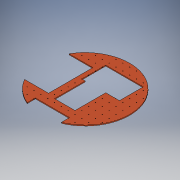
# Autodesk Inventor part: existing copper plate 1
Saved by Autodesk Inventor 2018 (Build 220112000, 112)
## iProperties
Created: 2018-11-02
Part Number: existing copper plate 1
Material: Copper
Document SubType Name: Modeling
Designer: freyja
Mass: 1197.4 g
Surface Area: 917.652 cm^2
Volume: 133.937 cm^3
Density: 8.94 g/cm^3
Appearance: Copper - Satin
Author: freyja
Autodesk Inventor part; units mm, degrees
ref_plane "YZ Plane" through (0, 0, 0) normal (1, 0, 0) x (0, 1, 0)
ref_plane "XZ Plane" through (0, 0, 0) normal (0, 1, 0) x (-1, 0, 0)
ref_plane "XY Plane" through (0, 0, 0) normal (0, 0, 1) x (1, 0, 0)
sketch "Sketch1" plane through (0, 0, 0) normal (0, 1, 0) x (-1, 0, 0)
  circle A0 centre (0, 0) radius 165.1
  dimension "d0" = 330.2
  constraints: 1 centre point, 1 coincident
  measures "d0" diameter of A0
extrude "Extrusion1" add sketch "Sketch1" along normal blind 3.175
sketch "Sketch2" plane through (0, 3.175, 0) normal (0, 1, 0) x (1, 0, 0)
  line L0 (0, 0) -> (-12.7, 0)
  line L1 (0, 0) -> (12.7, 0) construction
  circle A0 centre (0, 0) radius 165.1 projected
  dimension "d34" = 12.7
  dimension "d35" = 180
  constraints: 4 end point, 3 coincident, 2 horizontal, 1 collinear
  measures "d34" distance of L0.start L0.end
  measures "d35" angle of L0 L1
hole "Hole1" at (-12.7, 3.175, 0) direction (0, -1, 0) diameter 2.159 end through all
pattern_linear "Rectangular Pattern1" count 13 spacing 25.4 along (1, 0, 0) count 13 spacing 25.4 along (0, 0, 1) of "Hole1" first direction both ways yes second direction both ways yes
sketch "Sketch3" plane through (0, 3.175, 0) normal (0, 1, 0) x (1, 0, 0)
  circle A0 centre (0, 0) radius 165.1 projected
  line L0 (165.1, 0) -> (50.8, 0) construction
  line L1 (50.8, -88.9) -> (-25.4, -88.9)
  line L2 (-25.4, -88.9) -> (-25.4, 114.3)
  line L3 (-25.4, 114.3) -> (50.8, 114.3)
  line L4 (50.8, 114.3) -> (50.8, -88.9)
  line L5 (50.8, -88.9) -> (-25.4, 114.3) construction
  line L6 (-25.4, -88.9) -> (50.8, 114.3) construction
  line L7 (0, 165.1) -> (0, 114.3) construction
  line L8 (101.6, 25.4) -> (-38.1, 25.4)
  line L9 (-38.1, 25.4) -> (-38.1, 114.3)
  line L10 (-38.1, 114.3) -> (101.6, 114.3)
  line L11 (101.6, 114.3) -> (101.6, 25.4)
  line L12 (-25.4, 114.3) -> (-38.1, 114.3) construction
  line L13 (-25.4, -88.9) -> (-25.4, -121.92) construction
  line L14 (-63.5, -198.12) -> (63.5, -198.12)
  line L15 (63.5, -198.12) -> (63.5, -121.92)
  line L16 (63.5, -121.92) -> (-63.5, -121.92)
  line L17 (-63.5, -121.92) -> (-63.5, -198.12)
  line L18 (0, 0) -> (0, -165.1) construction
  line L19 (0, -198.12) -> (0, -121.92)
  line L20 (-181.0808, -82.55) -> (-181.0808, 82.55)
  line L21 (-181.0808, 82.55) -> (-54.0808, 82.55)
  line L22 (-54.0808, 82.55) -> (-54.0808, -82.55)
  line L23 (-54.0808, -82.55) -> (-181.0808, -82.55)
  line L24 (-142.9808, 82.55) -> (-54.0808, 82.55)
  circle A1 centre (0, 0) radius 165.1 projected
  line L25 (-142.9808, -82.55) -> (-54.0808, -82.55)
  point P0 (12.7, 12.7)
  dimension "d16" = 114.3
  dimension "d17" = 76.2
  dimension "d18" = 203.2
  dimension "d19" = 50.8
  dimension "d20" = 139.7
  dimension "d21" = 88.9
  dimension "d22" = 12.7
  dimension "d23" = 33.02
  dimension "d24" = 127
  dimension "d25" = 76.2
  dimension "d26" = 165.1
  dimension "d27" = 127
  dimension "d28" = 88.9
  dimension "d30" = 88.9
  constraints: 52 end point, 8 parallel, 7 horizontal, 6 point on circle, 5 perpendicular, 5 point on line, 4 midpoint, 4 vertical, 3 collinear, 2 line through centre
  measures "d16" distance of L0.start L0.end
  measures "d17" distance of L1.start L1.end
  measures "d18" distance of L1.end L2.end
  measures "d19" distance of L7.start L7.end
  measures "d20" distance of L9.end L10.end
  measures "d21" distance of L8.end L9.end
  measures "d22" distance of L2.end L12.end
  measures "d23" distance of L1.end L13.end
  measures "d24" distance of L16.end L15.end
  measures "d25" distance of L15.end L14.end
  measures "d26" distance of L20.start L20.end
  measures "d27" distance of L20.end L21.end
  measures "d28" distance of L21.end L24.start
  measures "d30" distance of L22.end L25.start
extrude "Extrusion2" cut sketch "Sketch3" against normal blind 3.175 contours L21 L22 L23 A0 | L15 L14 L19 A0 | A0 L19 L16 L15 | L19 L14 L17 A0 | A0 L17 L16 L19 | L1 L2 L8 L4 | L8 L2 L3 L4 | L4 L10 L11 L8 | L8 L9 L10 L2
body "Solid1"
